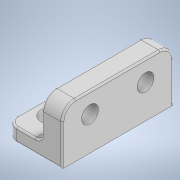
# Autodesk Inventor part: Wlan-antennen-halter
Saved by Autodesk Inventor 2021.3 (Build 253353010, 353A)
## iProperties
Created: 2021-08-30
Part Number: Wlan-antennen-halter
Material: Generisch
Document SubType Name: Modeling
Designer: Markus
Density: 1 g/cm^3
Appearance: Vorgabe
Author: Markus
Autodesk Inventor part; units mm, degrees
ref_plane "YZ Plane" through (0, 0, 0) normal (1, 0, 0) x (0, 1, 0)
ref_plane "XZ Plane" through (0, 0, 0) normal (0, 1, 0) x (-1, 0, 0)
ref_plane "XY Plane" through (0, 0, 0) normal (0, 0, 1) x (1, 0, 0)
sketch "Skizze1" plane through (0, 0, 0) normal (0, 1, 0) x (-1, 0, 0)
  line L0 (7.5, 16.5) -> (0, 16.5)
  line L1 (0, 16.5) -> (0, -16.5)
  line L2 (0, -16.5) -> (7.5, -16.5)
  line L3 (10.5, -13.5) -> (10.5, 13.5)
  circle A0 centre (5.25, 8.25) radius 3.25
  line L4 (10.5, 0) -> (0, 0) construction
  circle A1 centre (5.25, -8.25) radius 3.25
  arc A2 (10.5, 13.5) -> (7.5, 16.5) centre (7.5, 13.5) ccw
  arc A3 (7.5, -16.5) -> (10.5, -13.5) centre (7.5, -13.5) ccw
  point P0 (5.25, 0)
  dimension "d0" = 2
  dimension "d1" = 6.5
  dimension "d2" = 5
  dimension "d3" = 10
  dimension "d4" = 3
  constraints: 10 end point, 4 centre point, 4 point on circle, 4 tangent, 3 midpoint, 2 coincident, 2 parallel, 1 equal radius, 1 horizontal, 1 perpendicular, 1 vertical alignment, 1 other
  measures "d0" distance edge to line of A0 L3
  measures "d1" diameter of A0
  measures "d2" distance edge to line of A0 L0
  measures "d4" radius of A2
extrude "Extrusion1" add sketch "Skizze1" along normal blind 4
sketch "Skizze3" plane through (0, 0, 16.5) normal (1, 0, 0) x (0, 0, -1)
  line L0 (0, 0) -> (33, 0) projected
  line L1 (33, 0) -> (0, 0)
  line L2 (0, 0) -> (0, 16)
  line L3 (0, 16) -> (33, 16)
  line L4 (33, 16) -> (33, 0)
  point P0 (16.5, 0)
  point P1 (33, 4)
  dimension "d21" = 12
  constraints: 8 end point, 3 parallel, 1 horizontal, 1 perpendicular, 1 point on line
  measures "d21" distance from line of L3 point (33, 4)
extrude "Extrusion2" add sketch "Skizze3" along normal blind 6
sketch "Skizze4" plane through (0, 0, 16.5) normal (-1, 0, 0) x (0, 0, 1)
  point P0 (-16.5, 0)
sketch "Skizze5" plane through (0, 0, 16.5) normal (-1, 0, 0) x (0, 0, 1)
  line L0 (0, 4) -> (-33, 4) projected
  line L1 (0, 16) -> (0, 4) projected
  line L2 (-33, 16) -> (0, 16) projected
  line L3 (-33, 4) -> (-33, 16) projected
  line L4 (-33, 16) -> (0, 16) construction
  line L5 (-16.5, 16) -> (-16.5, 4) construction
  line L6 (-30, 4) -> (-3, 4) construction
  line L7 (-16.5, 10) -> (-33, 10) construction
  line L8 (-33, 0) -> (-33, 16) construction
  point P0 (-16.5, 0)
  point P1 (-24.75, 10)
  point P2 (-8.25, 10)
  point P3 (-24.75, 10)
  constraints: 4 end point, 4 midpoint, 1 coincident, 1 horizontal alignment, 1 perpendicular, 1 point on line, 1 symmetric about line
hole "Bohrung1" at (0, 10, 8.25) at (0, 10, -8.25) direction (1, 0, 0) diameter 5 end through all countersink diameter 8.6 countersink angle 90
fillet "Rundung1" radius 2 1 edges at (0, 4, 0)
fillet "Rundung2" radius 4 2 edges at (3, 16, 16.5) (3, 16, -16.5)
fillet "Rundung3" radius 0.5 22 edges at (6, 14.8284, 15.3284) (6, 16, 0) (6, 14.8284, -15.3284) (6, 6, -16.5) (6, 6, 16.5) (-9.6213, 0, 15.6213) (-10.5, 0, 0) (-9.6213, 0, -15.6213) (-0.75, 0, -16.5) (-0.75, 0, 16.5) (0, 9, 16.5) (-0.5858, 4.5858, 16.5) (-4.75, 4, 16.5) (-9.6213, 4, 15.6213) (-10.5, 4, 0) (-9.6213, 4, -15.6213) (-4.75, 4, -16.5) (-0.5858, 4.5858, -16.5) (0, 9, -16.5) (0, 14.8284, -15.3284) (0, 16, 0) (0, 14.8284, 15.3284)
sketch "Skizze7" plane through (0, 4, 0) normal (0, 1, 0) x (1, 0, 0)
  circle A0 centre (-5.25, -8.25) radius 3.25 projected
  circle A1 centre (-5.25, 8.25) radius 3.25 projected
  circle A2 centre (-5.25, -8.25) radius 5.25
  circle A3 centre (-5.25, 8.25) radius 5.25
  point P0 (0, 0)
  point P1 (-2, -8.25)
  point P2 (-2, 8.25)
  dimension "d32" = 2
  constraints: 2 centre point, 2 horizontal alignment, 1 equal radius
extrude "Extrusion3" cut sketch "Skizze7" along normal up to surface (12 mm away)
